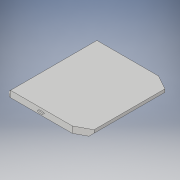
# Autodesk Inventor part: Moto G3 Phone Case Back
Saved by Autodesk Inventor 2019 (Build 230136000, 136)
## iProperties
Created: 2018-12-30
Part Number: Moto G3 Phone Case Back
Material: Generic
Document SubType Name: Modeling
Designer: mrhftc
Density: 1 g/cm^3
Appearance: Default
Author: mrhftc
Autodesk Inventor part; units mm, degrees
ref_plane "YZ Plane" through (0, 0, 0) normal (1, 0, 0) x (0, 1, 0)
ref_plane "XZ Plane" through (0, 0, 0) normal (0, 1, 0) x (-1, 0, 0)
ref_plane "XY Plane" through (0, 0, 0) normal (0, 0, 1) x (1, 0, 0)
sketch "Sketch1" plane through (0, 0, 0) normal (0, 1, 0) x (-1, 0, 0)
  line L0 (67.8505, 69.4133) -> (67.8505, -11.5697)
  line L1 (67.8505, -11.5697) -> (6.8505, -11.5697)
  line L2 (6.8505, -11.5697) -> (-6.5145, -4.1373)
  line L3 (-6.5145, -4.1373) -> (-6.5145, 62.3267)
  line L4 (-6.5145, 62.3267) -> (6.8505, 69.4133)
  line L5 (6.8505, 69.4133) -> (67.8505, 69.4133)
  constraints: 12 end point, 1 parallel, 1 perpendicular, 1 vertical
extrude "Extrusion1" add sketch "Sketch1" along normal blind 6
sketch "Sketch2" plane through (-6.8505, 0, -11.5697) normal (0, 0, -1) x (-1, 0, 0)
  line L0 (0, 0) -> (0, 6) construction
  ellipse E0 centre (28.92, 3) end of major axis (31.716, 3) minor radius 0.841
  line L1 (-13.365, 0) -> (-13.365, 6) construction
  point P0 (-6.8505, 0)
  dimension "d9" = 2.796
  dimension "d12" = 0.841
  dimension "d11" = 28.92
  constraints: 2 other
  measures "d11" distance from line of L0 point (28.92, 3)
extrude "Extrusion2" add sketch "Sketch2" along normal blind 1.125
sketch "Sketch3" plane through (-67.8505, 0, 69.4133) normal (0, 0, 1) x (1, 0, 0)
  ellipse E0 centre (32.08, 3) end of major axis (34.876, 3) minor radius 0.841 construction
  ellipse E1 centre (32.08, 3) end of major axis (29.284, 3) minor radius 0.841
  point P0 (67.8505, 0)
  constraints: 1 coincident, 3 other
extrude "Extrusion3" add sketch "Sketch3" along normal blind 1.125
chamfer "Chamfer1" distance 3.175 angle 45 1 edges at (-67.8505, 6, 28.9218)
fillet "Fillet1" radius 3.175 3 edges at (-67.8505, 0, 28.9218) (-67.8505, 1.4125, -11.5697) (-67.8505, 1.4125, 69.4133)
chamfer "Chamfer2" distance 3.175 angle 45 1 edges at (6.5145, 0, 29.0947)
body "Solid1"
